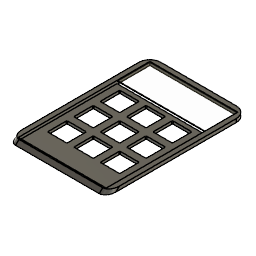
top (Autodesk Fusion 360 design; units mm, degrees)
part number: 2026-06-01-16-41-10-771
Autodesk Fusion 360 part; units mm, degrees
sketch "plate-2026-06-01T11_12_08.980Z" plane through (0, 0, 0) normal (0, 0, 1) x (1, 0, 0)
  line L0 (-14.2555, 38.7797) -> (-1.2555, 38.7797)
  line L1 (-14.2555, 24.7797) -> (-1.2555, 24.7797)
  line L2 (-14.7555, 38.2797) -> (-14.7555, 25.2797)
  line L3 (-0.7555, 38.2797) -> (-0.7555, 25.2797)
  arc A0 (-14.2555, 38.7797) -> (-14.7555, 38.2797) centre (-14.2555, 38.2797) ccw
  arc A1 (-0.7555, 38.2797) -> (-1.2555, 38.7797) centre (-1.2555, 38.2797) ccw
  arc A2 (-14.7555, 25.2797) -> (-14.2555, 24.7797) centre (-14.2555, 25.2797) ccw
  arc A3 (-1.2555, 24.7797) -> (-0.7555, 25.2797) centre (-1.2555, 25.2797) ccw
  line L4 (4.7945, 38.7797) -> (17.7945, 38.7797)
  line L5 (4.7945, 24.7797) -> (17.7945, 24.7797)
  line L6 (4.2945, 38.2797) -> (4.2945, 25.2797)
  line L7 (18.2945, 38.2797) -> (18.2945, 25.2797)
  arc A4 (4.7945, 38.7797) -> (4.2945, 38.2797) centre (4.7945, 38.2797) ccw
  arc A5 (18.2945, 38.2797) -> (17.7945, 38.7797) centre (17.7945, 38.2797) ccw
  arc A6 (4.2945, 25.2797) -> (4.7945, 24.7797) centre (4.7945, 25.2797) ccw
  arc A7 (17.7945, 24.7797) -> (18.2945, 25.2797) centre (17.7945, 25.2797) ccw
  line L8 (23.8445, 38.7797) -> (36.8445, 38.7797)
  line L9 (23.8445, 24.7797) -> (36.8445, 24.7797)
  line L10 (23.3445, 38.2797) -> (23.3445, 25.2797)
  line L11 (37.3445, 38.2797) -> (37.3445, 25.2797)
  arc A8 (23.8445, 38.7797) -> (23.3445, 38.2797) centre (23.8445, 38.2797) ccw
  arc A9 (37.3445, 38.2797) -> (36.8445, 38.7797) centre (36.8445, 38.2797) ccw
  arc A10 (23.3445, 25.2797) -> (23.8445, 24.7797) centre (23.8445, 25.2797) ccw
  arc A11 (36.8445, 24.7797) -> (37.3445, 25.2797) centre (36.8445, 25.2797) ccw
  line L12 (-14.2555, 19.7297) -> (-1.2555, 19.7297)
  line L13 (-14.2555, 5.7297) -> (-1.2555, 5.7297)
  line L14 (-14.7555, 19.2297) -> (-14.7555, 6.2297)
  line L15 (-0.7555, 19.2297) -> (-0.7555, 6.2297)
  arc A12 (-14.2555, 19.7297) -> (-14.7555, 19.2297) centre (-14.2555, 19.2297) ccw
  arc A13 (-0.7555, 19.2297) -> (-1.2555, 19.7297) centre (-1.2555, 19.2297) ccw
  arc A14 (-14.7555, 6.2297) -> (-14.2555, 5.7297) centre (-14.2555, 6.2297) ccw
  arc A15 (-1.2555, 5.7297) -> (-0.7555, 6.2297) centre (-1.2555, 6.2297) ccw
  line L16 (4.7945, 19.7297) -> (17.7945, 19.7297)
  line L17 (4.7945, 5.7297) -> (17.7945, 5.7297)
  line L18 (4.2945, 19.2297) -> (4.2945, 6.2297)
  line L19 (18.2945, 19.2297) -> (18.2945, 6.2297)
  arc A16 (4.7945, 19.7297) -> (4.2945, 19.2297) centre (4.7945, 19.2297) ccw
  arc A17 (18.2945, 19.2297) -> (17.7945, 19.7297) centre (17.7945, 19.2297) ccw
  arc A18 (4.2945, 6.2297) -> (4.7945, 5.7297) centre (4.7945, 6.2297) ccw
  arc A19 (17.7945, 5.7297) -> (18.2945, 6.2297) centre (17.7945, 6.2297) ccw
  line L20 (23.8445, 19.7297) -> (36.8445, 19.7297)
  line L21 (23.8445, 5.7297) -> (36.8445, 5.7297)
  line L22 (23.3445, 19.2297) -> (23.3445, 6.2297)
  line L23 (37.3445, 19.2297) -> (37.3445, 6.2297)
  arc A20 (23.8445, 19.7297) -> (23.3445, 19.2297) centre (23.8445, 19.2297) ccw
  arc A21 (37.3445, 19.2297) -> (36.8445, 19.7297) centre (36.8445, 19.2297) ccw
  arc A22 (23.3445, 6.2297) -> (23.8445, 5.7297) centre (23.8445, 6.2297) ccw
  arc A23 (36.8445, 5.7297) -> (37.3445, 6.2297) centre (36.8445, 6.2297) ccw
  line L24 (-14.2555, 0.6797) -> (-1.2555, 0.6797)
  line L25 (-14.2555, -13.3203) -> (-1.2555, -13.3203)
  line L26 (-14.7555, 0.1797) -> (-14.7555, -12.8203)
  line L27 (-0.7555, 0.1797) -> (-0.7555, -12.8203)
  arc A24 (-14.2555, 0.6797) -> (-14.7555, 0.1797) centre (-14.2555, 0.1797) ccw
  arc A25 (-0.7555, 0.1797) -> (-1.2555, 0.6797) centre (-1.2555, 0.1797) ccw
  arc A26 (-14.7555, -12.8203) -> (-14.2555, -13.3203) centre (-14.2555, -12.8203) ccw
  arc A27 (-1.2555, -13.3203) -> (-0.7555, -12.8203) centre (-1.2555, -12.8203) ccw
  line L28 (4.7945, 0.6797) -> (17.7945, 0.6797)
  line L29 (4.7945, -13.3203) -> (17.7945, -13.3203)
  line L30 (4.2945, 0.1797) -> (4.2945, -12.8203)
  line L31 (18.2945, 0.1797) -> (18.2945, -12.8203)
  arc A28 (4.7945, 0.6797) -> (4.2945, 0.1797) centre (4.7945, 0.1797) ccw
  arc A29 (18.2945, 0.1797) -> (17.7945, 0.6797) centre (17.7945, 0.1797) ccw
  arc A30 (4.2945, -12.8203) -> (4.7945, -13.3203) centre (4.7945, -12.8203) ccw
  arc A31 (17.7945, -13.3203) -> (18.2945, -12.8203) centre (17.7945, -12.8203) ccw
  line L32 (23.8445, 0.6797) -> (36.8445, 0.6797)
  line L33 (23.8445, -13.3203) -> (36.8445, -13.3203)
  line L34 (23.3445, 0.1797) -> (23.3445, -12.8203)
  line L35 (37.3445, 0.1797) -> (37.3445, -12.8203)
  arc A32 (23.8445, 0.6797) -> (23.3445, 0.1797) centre (23.8445, 0.1797) ccw
  arc A33 (37.3445, 0.1797) -> (36.8445, 0.6797) centre (36.8445, 0.1797) ccw
  arc A34 (23.3445, -12.8203) -> (23.8445, -13.3203) centre (23.8445, -12.8203) ccw
  arc A35 (36.8445, -13.3203) -> (37.3445, -12.8203) centre (36.8445, -12.8203) ccw
  line L36 (-23.3335, 69.1387) -> (47.1165, 69.1387)
  line L37 (47.1165, 69.1387) -> (47.1165, -32.8613)
  line L38 (47.1165, -32.8613) -> (-23.3335, -32.8613)
  line L39 (-23.3335, -32.8613) -> (-23.3335, 69.1387)
  line L40 (-19.8335, 65.6387) -> (43.6165, 65.6387)
  line L41 (43.6165, 65.6387) -> (43.6165, -29.3613)
  line L42 (43.6165, -29.3613) -> (-19.8335, -29.3613)
  line L43 (-19.8335, -29.3613) -> (-19.8335, 65.6387)
  line L44 (-19.8335, 65.6387) -> (43.6165, 65.6387)
  line L45 (43.6165, 65.6387) -> (43.6165, 42.0048)
  line L46 (43.6165, 42.0048) -> (-19.8335, 42.0048)
  line L47 (-19.8335, 42.0048) -> (-19.8335, 65.6387)
  dimension "d1" = 70.45
  dimension "d2" = 102
  dimension "d3" = 9.772
  dimension "d4" = 19.541
  dimension "d7" = 3.5
  dimension "d8" = 3.5
  dimension "d9" = 3.5
  dimension "d10" = 3.5
  constraint horizontal L36
  constraint vertical L37
  constraint horizontal L38
  constraint vertical L39
  constraint horizontal L40
  constraint vertical L41
  constraint horizontal L42
  constraint vertical L43
  constraint horizontal L44
  constraint vertical L45
  constraint horizontal L46
  constraint vertical L47
  constraint coincident L41 L45.end
  measures "d1" distance of L37 L39
  measures "d2" distance of L36 L38
  measures "d3" distance of L35 L37
  measures "d4" distance of L33 L38
  measures "d7" distance of L36 L40
  measures "d8" distance of L39 L43
  measures "d9" distance of L37 L41
  measures "d10" distance of L38 L42
extrude "Extrude1" add sketch "plate-2026-06-01T11_12_08.980Z" along normal blind 2 contours L36 L37 L38 L39 | L40 L41 L43 L44 L45 L46 L47 | L41 L42 L43 L46 makes body 1
extrude "Extrude2" cut sketch "plate-2026-06-01T11_12_08.980Z" along normal blind 7 contours L40 L41 L43 L44 L45 L46 L47 bodies 1
extrude "Extrude3" add sketch "plate-2026-06-01T11_12_08.980Z" along normal blind 4 contours L36 L37 L38 L39 bodies 1
extrude "Extrude4" cut sketch "plate-2026-06-01T11_12_08.980Z" along normal blind 1.5 contours L36 L37 L38 L39 bodies 1
fillet "Fillet1" radius 8 2 edges at (-23.3335, 69.1387, 2.75) (47.1165, 69.1387, 2.75) on bodies 1
sketch "Sketch2" plane through (0, -32.8613, 0) normal (0, -1, 0) x (1, 0, 0)
  line L0 (47.1165, 4) -> (-23.3335, 4)
  line L1 (-23.3335, 1.5) -> (47.1165, 1.5)
  line L2 (-23.3335, 4) -> (47.1165, 4)
  line L3 (47.1165, 1.5) -> (47.1165, 4)
  line L4 (-23.3335, 4) -> (-23.3335, 1.5)
  constraint coincident L0.end L2.start
  constraint coincident L0.start L2.end
chamfer "Chamfer1" distance 2.5 angle 45 1 edges at (11.8915, -32.8613, 4) on bodies 1
fillet "Fillet2" radius 5 2 edges at (-23.3335, -31.6113, 2.75) (47.1165, -31.6113, 2.75) on bodies 1
extrude "Extrude5" add sketch "plate-2026-06-01T11_12_08.980Z" along normal blind 4 separate body contours L40 L41 L43 L44 L45 L46 L47 makes body 2
extrude "Extrude6" cut sketch "plate-2026-06-01T11_12_08.980Z" along normal blind 3.5 contours L40 L41 L43 L44 L45 L46 L47 bodies 2
